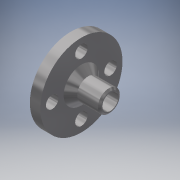
# Autodesk Inventor part: Flange 1 in
Saved by Autodesk Inventor 2016 (Build 200138000, 138)
## iProperties
Created: 2018-11-07
Part Number: Flange 1 in
Material: ASTM A105 Gr.B
Document SubType Name: Modeling
Designer: Wijaya
Mass: 1553.05 g
Surface Area: 404.269 cm^2
Volume: 197.841 cm^3
Density: 7.85 g/cm^3
Appearance: Semi-Polished
Author: Wijaya
Autodesk Inventor part; units mm, degrees
note: some values were not read from the file. Chosen so that the rebuilt part matches the saved one: direction of "Hole1".
ref_plane "YZ Plane" through (0, 0, 0) normal (1, 0, 0) x (0, 1, 0)
ref_plane "XZ Plane" through (0, 0, 0) normal (0, 1, 0) x (-1, 0, 0)
ref_plane "XY Plane" through (0, 0, 0) normal (0, 0, 1) x (1, 0, 0)
sketch "Sketch1" plane through (0, 0, 0) normal (0, 0, 1) x (1, 0, 0)
  line L0 (0, 0) -> (93, 0)
  line L1 (0, 12.15) -> (0, 27)
  line L2 (0, 27) -> (2, 27)
  line L3 (2, 27) -> (2, 62.5)
  line L4 (2, 62.5) -> (17.9, 62.5)
  line L5 (17.9, 62.5) -> (17.9, 27)
  line L6 (17.9, 27) -> (28.2, 16.7)
  line L7 (28.2, 16.7) -> (59.7364, 16.7)
  line L8 (59.7364, 16.7) -> (62, 13.75)
  line L9 (62, 13.75) -> (62, 12.15)
  line L10 (62, 12.15) -> (0, 12.15)
  point P0 (0, 19.575)
  dimension "d5" = 125
  dimension "d6" = 54
  dimension "d7" = 2
  dimension "d8" = 15.9
  dimension "d9" = 45
  dimension "d10" = 60
  dimension "d27" = 37.5
  dimension "d28" = 24.3
  dimension "d29" = 33.4
  dimension "d30" = 1.6
  constraints: 22 end point, 5 perpendicular, 2 parallel, 1 horizontal, 1 midpoint, 1 point on line, 1 vertical alignment
  measures "d5" diameter of L4 L0
  measures "d6" diameter of L2 L0
  measures "d7" distance of L1.end L2.end
  measures "d8" distance of L3.end L4.end
  measures "d9" angle of L7 L6
  measures "d10" distance from line of L8.end L3
  measures "d27" angle of L9 L8
  measures "d28" diameter of L10 L0
  measures "d29" diameter of L7 L0
  measures "d30" distance of L8.end L9.end
revolve "Revolution1" add sketch "Sketch1" angle 360 about axis through (0, 0, 0) along (1, 0, 0)
sketch "Sketch3" plane through (2, 0, 0) normal (-1, 0, 0) x (0, 0, 1)
  point P0 (0, 0)
  point P1 (0, 44.45)
  dimension "d16" = 44.45
  constraints: 1 vertical alignment
  measures "d16" distance of point (0, 0) point (0, 44.45)
hole "Hole1" at (2, 44.45, 0) direction (1, 0, 0) diameter 19.05 end up to surface
pattern_circular "Circular Pattern1" count 4 over 360 about axis through (9.95, 0, 0) along (1, 0, 0) of "Hole1"
body "Solid1"
